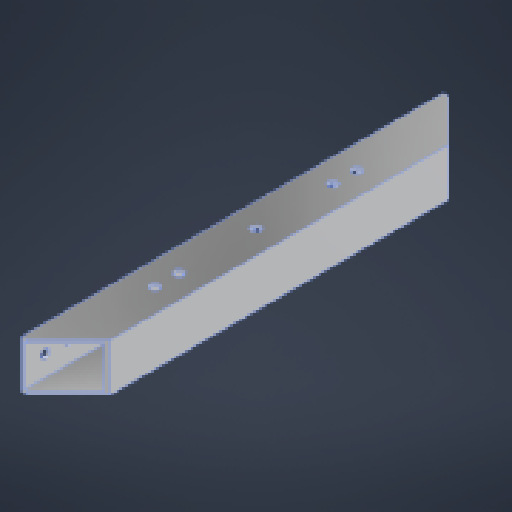
# Autodesk Inventor part: climber-main-arm
Saved by Autodesk Inventor 2025.1 (Build 291241020, 241B)
## iProperties
ILogicPurgeVersion: 0.0.0.0
OnSaveVersion: 2.2.20.20
RuleStatus: InUse
Category: _
Manager: _
Created: 2025-03-18
Part Number: climber-main-arm
Checked By: 0002334344
Engr Approved By: R
User Status: Work In Process
Material: Aluminum 6061
Description: TEMPLATE,TUBING
Document SubType Name: Modeling
Mfg Approved By: Stephen.Oerton
Designer: mathe
Mass: 62.2196 g
Surface Area: 293.346 cm^2
Volume: 23.0443 cm^3
Density: 2.7 g/cm^3
Appearance: Aluminum - Flat
CN_MASS: 2.01
PTC_WM_ITERATION: 1
PTC_WM_ORGANIZATION_ID: CLWC
PTC_WM_LIFECYCLE: CLWC_CAD_LC
CL_runCount: 0
Length: 0.19" WALL X 2" X 2" X 300.0 mm Lg
ModelCat: Tube
FIRST_DESCRIPTION: _
SECOND_DESCRIPTION: _
THIRD_DESCRIPTION: _
CN_SERVICEABLE: _
Subject: _
Author: mathe
Keywords: -
Revision Number: A
Autodesk Inventor part; units mm, degrees
ref_plane "YZ Plane" through (0, 0, 0) normal (1, 0, 0) x (0, 1, 0)
ref_plane "XZ Plane" through (0, 0, 0) normal (0, 1, 0) x (-1, 0, 0)
ref_plane "XY Plane" through (0, 0, 0) normal (0, 0, 1) x (1, 0, 0)
sketch "Sketch1" plane through (0, 0, 0) normal (0, 0, 1) x (1, 0, 0)
  line L0 (-12.7, 12.7) -> (12.7, 12.7)
  line L1 (12.7, 12.7) -> (12.7, -12.7)
  line L2 (12.7, -12.7) -> (-12.7, -12.7)
  line L3 (-12.7, -12.7) -> (-12.7, 12.7)
  line L4 (0, 0) -> (0, -12.7) construction
  line L5 (-17.78, 0) -> (17.78, 0) construction
  dimension "d10" = 12.7
  dimension "RotateAngle" = 90
  constraints: 10 end point, 2 parallel, 1 horizontal alignment, 1 midpoint, 1 perpendicular, 1 vertical alignment, 1 other
  measures "d10" distance from line of L4.start L0
  measures "RotateAngle" angle of L4 L5
extrude "Extrusion1" add sketch "Sketch1" along normal mid plane 225.425
shell "Shell1" thickness 1.5875 removed faces 2 at (-4.2333, -4.2333, 112.7125) at (-4.2333, -4.2333, -112.7125)
feature "TaperEdge1-YZ" [suppressed]
feature "TaperEdge2-YZ" [suppressed]
feature "TaperEdge1-XZ" [suppressed]
feature "TaperEdge2-XZ" [suppressed]
sketch "Sketch4" plane through (0, -63.5, 762) normal (1, 0, 0) x (0, 0, -1)
  line L0 (254.5, 63.5) -> (534.5, 63.5) construction
  line L1 (254.5, 26) -> (534.5, 26)
  line L2 (534.5, 101) -> (254.5, 101)
  arc A0 (254.5, 101) -> (254.5, 26) centre (254.5, 63.5) ccw
  arc A1 (534.5, 26) -> (534.5, 101) centre (534.5, 63.5) ccw
  line L3 (989.5, 63.5) -> (1269.5, 63.5) construction
  line L4 (989.5, 26) -> (1269.5, 26)
  line L5 (1269.5, 101) -> (989.5, 101)
  arc A2 (989.5, 101) -> (989.5, 26) centre (989.5, 63.5) ccw
  arc A3 (1269.5, 26) -> (1269.5, 101) centre (1269.5, 63.5) ccw
  point P0 (762, 63.5)
  point P1 (394.5, 63.5)
  point P2 (1129.5, 63.5)
  dimension "d24" = 280
  dimension "d25" = 75
  dimension "d27" = 1015
  dimension "d28" = 507.5
  constraints: 16 end point, 8 point on circle, 8 tangent, 4 centre point, 2 midpoint, 2 parallel, 2 point on line, 1 collinear, 1 equal radius, 1 horizontal, 1 horizontal alignment
  measures "d24" distance of L0.start L0.end
  measures "d25" distance between parallel lines of L1 L2
  measures "d27" distance of L3.end L0.start
  measures "d28" distance of point (762, 63.5) L0.start
extrude "ForkSlots" [suppressed]
sketch "Sketch6" plane through (-12.7, 12.7, 112.7125) normal (0, 1, 0) x (1, 0, 0)
  line L0 (12.7, 112.7125) -> (12.7, 153.9875)
  line L1 (12.7, 153.9875) -> (12.7, 166.6875)
  line L2 (12.7, 112.7125) -> (-0.1137, 112.7125) construction
  line L3 (12.7, 112.7125) -> (12.7, 71.4375)
  line L4 (12.7, 71.4375) -> (12.7, 58.7375)
  dimension "d46" = 41.275
  dimension "d47" = 12.7
  constraints: 10 end point, 6 coincident, 4 symmetric about line, 2 vertical, 1 horizontal
  measures "d46" distance of L0.start L0.end
  measures "d47" distance of L0.end L1.end
hole "Hole2" at (0, 12.7, 0) at (0, 12.7, -41.275) at (0, 12.7, -53.975) at (0, 12.7, 53.975) at (0, 12.7, 41.275) direction (0, -1, 0) diameter 5.1 end through all
sketch "Sketch7" plane through (-12.7, -12.7, 112.7125) normal (0, -1, 0) x (1, 0, 0)
  circle A0 centre (12.7, -71.4375) radius 2.55 projected
  circle A1 centre (12.7, -58.7375) radius 2.55 projected
  circle A2 centre (12.7, -166.6875) radius 2.55 projected
  circle A3 centre (12.7, -153.9875) radius 2.55 projected
  circle A4 centre (12.7, -112.7125) radius 2.55 projected
  line L0 (25.4, 0) -> (0, 0) projected
  line L1 (0, 0) -> (0, -225.425) projected
  line L2 (0, -225.425) -> (25.4, -225.425) projected
  line L3 (25.4, 0) -> (25.4, -225.425) projected
  line L4 (0, -225.425) -> (3.175, -225.425)
  line L5 (3.175, -225.425) -> (25.4, -203.2)
  line L6 (3.175, -225.425) -> (34.6059, -225.425) construction
  line L7 (12.7, -112.7125) -> (0, -112.7125) construction
  line L8 (3.175, 0) -> (25.4, -22.225)
  point P0 (3.175, 0)
  dimension "d55" = 3.175
  dimension "d56" = 45
  constraints: 10 end point, 2 point on line, 2 symmetric about line, 1 equal length, 1 horizontal, 1 midpoint
  measures "d55" distance of L1.end L4.end
  measures "d56" angle of L6 L5
extrude "Extrusion5" cut sketch "Sketch7" against normal up to surface (25.4 mm away) contours L3 L8 L0 | L3 L2 L5
sketch "Sketch8" plane through (-12.7, -12.7, 112.7125) normal (-1, 0, 0) x (0, 0, 1)
  line L0 (0, 0) -> (0, 25.4) projected
  line L1 (-225.425, 25.4) -> (0, 25.4) projected
  line L2 (-225.425, 25.4) -> (-225.425, 0) projected
  line L3 (0, 0) -> (-225.425, 0) projected
  line L4 (-225.425, 25.4) -> (-225.425, 0) projected
  line L5 (-225.425, 12.7) -> (-212.725, 12.7)
  circle A0 centre (-214.3125, 12.7) radius 2.5527 projected
  point P0 (-112.7125, 12.7)
  point P1 (-201.6125, 12.7)
  point P2 (-201.6125, 12.7)
  point P3 (-188.9125, 12.7)
  point P4 (-188.9125, 12.7)
  point P5 (-176.2125, 12.7)
  point P6 (-176.2125, 12.7)
  point P7 (-163.5125, 12.7)
  point P8 (-163.5125, 12.7)
  point P9 (-150.8125, 12.7)
  point P10 (-150.8125, 12.7)
  point P11 (-138.1125, 12.7)
  point P12 (-138.1125, 12.7)
  point P13 (-125.4125, 12.7)
  point P14 (-125.4125, 12.7)
  point P15 (-112.7125, 12.7)
  point P16 (-112.7125, 12.7)
  point P17 (-100.0125, 12.7)
  point P18 (-100.0125, 12.7)
  point P19 (-87.3125, 12.7)
  point P20 (-87.3125, 12.7)
  point P21 (-74.6125, 12.7)
  point P22 (-74.6125, 12.7)
  point P23 (-61.9125, 12.7)
  point P24 (-61.9125, 12.7)
  point P25 (-49.2125, 12.7)
  point P26 (-49.2125, 12.7)
  point P27 (-36.5125, 12.7)
  point P28 (-36.5125, 12.7)
  point P29 (-23.8125, 12.7)
  point P30 (-23.8125, 12.7)
  point P31 (-11.1125, 12.7)
  point P32 (-11.1125, 12.7)
  dimension "d62" = 12.7
  constraints: 17 coincident, 2 end point, 2 horizontal, 1 midpoint, 32 other
  measures "d62" distance of A0.centre point (-201.613, 12.7)
hole "Hole3" at (-12.7, 0, -101.6) at (-12.7, 0, -88.9) at (-12.7, 0, -76.2) at (-12.7, 0, -63.5) at (-12.7, 0, -50.8) at (-12.7, 0, -38.1) at (-12.7, 0, -25.4) at (-12.7, 0, -12.7) at (-12.7, 0, 0) at (-12.7, 0, 12.7) at (-12.7, 0, 25.4) at (-12.7, 0, 38.1) at (-12.7, 0, 50.8) at (-12.7, 0, 63.5) at (-12.7, 0, 76.2) at (-12.7, 0, 88.9) at (-12.7, 0, 101.6) direction (1, 0, 0) diameter 5.1 depth 8 tip angle 118
